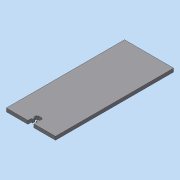
# Autodesk Inventor part: Y-Shafts-Holder_Side
Saved by Autodesk Inventor 2016 SP1 (Build 200210100, 210)
## iProperties
Created: 2016-01-21
Part Number: Y-Shafts-Holder_Side
Material: Generic
Document SubType Name: Modeling
Designer: Mohamed A.
Density: 1 g/cm^3
Appearance: Default
Author: Mohamed A.
Autodesk Inventor part; units mm, degrees
ref_plane "YZ Plane" through (0, 0, 0) normal (1, 0, 0) x (0, 1, 0)
ref_plane "XZ Plane" through (0, 0, 0) normal (0, 1, 0) x (-1, 0, 0)
ref_plane "XY Plane" through (0, 0, 0) normal (0, 0, 1) x (1, 0, 0)
sketch "Sketch1" plane through (0, 0, 0) normal (0, 0, 1) x (1, 0, 0)
  line L0 (-21.5, 51.7145) -> (21.5, 51.7145)
  line L1 (21.5, 51.7145) -> (21.5, -51.7145)
  line L2 (-21.5, -51.7145) -> (-21.5, 51.7145)
  line L3 (5.5, -51.7145) -> (5.5, -48.7145)
  line L4 (1.5, -46.7145) -> (2.65, -46.7145)
  line L5 (2.65, -46.7145) -> (2.65, -44.3145)
  line L6 (2.65, -44.3145) -> (1.5, -44.3145)
  line L7 (1.5, -44.3145) -> (1.5, -43.7145)
  line L8 (1.5, -43.7145) -> (-1.5, -43.7145)
  line L9 (-1.5, -43.7145) -> (-1.5, -44.3145)
  line L10 (-1.5, -44.3145) -> (-2.65, -44.3145)
  line L11 (-2.65, -44.3145) -> (-2.65, -46.7145)
  line L12 (-2.65, -46.7145) -> (-1.5, -46.7145)
  line L13 (-5.5, -48.7145) -> (-5.5, -51.7145)
  line L14 (1.5, -46.7145) -> (1.5, -48.7145)
  line L15 (1.5, -48.7145) -> (5.5, -48.7145)
  line L16 (-1.5, -46.7145) -> (-1.5, -48.7145)
  line L17 (-1.5, -48.7145) -> (-5.5, -48.7145)
  line L18 (21.5, -51.7145) -> (13.5, -51.7145)
  line L19 (-5.5, -51.7145) -> (-21.5, -51.7145)
  line L20 (-30.1, 0) -> (30.1, 0) construction
  line L21 (0, -72.4008) -> (0, 72.4004) construction
  line L22 (13.5, 44.7145) -> (13.5, 51.7145) projected
  line L23 (13.5, 51.7145) -> (10.5, 51.7145) projected
  line L24 (10.5, 44.7145) -> (10.5, 51.7145) projected
  line L25 (13.5, 44.7145) -> (10.5, 44.7145) projected
  line L26 (13.5, -4.1443) -> (13.5, 18.7145) projected
  line L27 (13.5, 18.7145) -> (10.5, 18.7145) projected
  line L28 (10.5, -4.1443) -> (10.5, 18.7145) projected
  line L29 (13.5, -4.1443) -> (10.5, -4.1443) projected
  line L30 (13.5, -51.7149) -> (13.5, -30.1443) projected
  line L31 (13.5, -30.1443) -> (10.5, -30.1443) projected
  line L32 (10.5, -51.7149) -> (10.5, -30.1443) projected
  line L33 (13.5, -51.7149) -> (10.5, -51.7149) projected
  line L34 (16.5, 41.7145) -> (16.5, 34.3645) projected
  line L35 (16.5, 41.7145) -> (13.5, 41.7145) projected
  line L36 (13.5, 34.3645) -> (13.5, 41.7145) projected
  line L37 (16.5, 34.3645) -> (13.5, 34.3645) projected
  line L38 (16.5, 29.0645) -> (16.5, 21.7145) projected
  line L39 (16.5, 29.0645) -> (13.5, 29.0645) projected
  line L40 (13.5, 21.7145) -> (13.5, 29.0645) projected
  line L41 (16.5, 21.7145) -> (13.5, 21.7145) projected
  line L42 (16.5, -7.1443) -> (16.5, -14.4943) projected
  line L43 (16.5, -7.1443) -> (13.5, -7.1443) projected
  line L44 (13.5, -14.4943) -> (13.5, -7.1443) projected
  line L45 (16.5, -14.4943) -> (13.5, -14.4943) projected
  line L46 (16.5, -19.7943) -> (16.5, -27.1443) projected
  line L47 (16.5, -19.7943) -> (13.5, -19.7943) projected
  line L48 (13.5, -27.1443) -> (13.5, -19.7943) projected
  line L49 (16.5, -27.1443) -> (13.5, -27.1443) projected
  line L50 (-13.5, -19.7943) -> (-13.5, -27.1443) projected
  line L51 (-13.5, -19.7943) -> (-16.5, -19.7943) projected
  line L52 (-16.5, -27.1443) -> (-16.5, -19.7943) projected
  line L53 (-13.5, -27.1443) -> (-16.5, -27.1443) projected
  line L54 (-13.5, -7.1443) -> (-13.5, -14.4943) projected
  line L55 (-13.5, -7.1443) -> (-16.5, -7.1443) projected
  line L56 (-16.5, -14.4943) -> (-16.5, -7.1443) projected
  line L57 (-13.5, -14.4943) -> (-16.5, -14.4943) projected
  line L58 (-13.5, 29.0645) -> (-13.5, 21.7145) projected
  line L59 (-13.5, 29.0645) -> (-16.5, 29.0645) projected
  line L60 (-16.5, 21.7145) -> (-16.5, 29.0645) projected
  line L61 (-13.5, 21.7145) -> (-16.5, 21.7145) projected
  line L62 (-13.5, 41.7145) -> (-13.5, 34.3645) projected
  line L63 (-13.5, 41.7145) -> (-16.5, 41.7145) projected
  line L64 (-16.5, 34.3645) -> (-16.5, 41.7145) projected
  line L65 (-13.5, 34.3645) -> (-16.5, 34.3645) projected
  line L66 (16.5, 34.3645) -> (13.5, 29.0645) construction
  line L67 (13.5, 34.3645) -> (16.5, 29.0645) construction
  line L68 (13.5, -14.4943) -> (16.5, -19.7943) construction
  line L69 (16.5, -14.4943) -> (13.5, -19.7943) construction
  line L70 (-13.5, -14.4943) -> (-16.5, -19.7943) construction
  line L71 (-16.5, -14.4943) -> (-13.5, -19.7943) construction
  line L72 (-13.5, 34.3645) -> (-16.5, 29.0645) construction
  line L73 (-16.5, 34.3645) -> (-13.5, 29.0645) construction
  circle A0 centre (-15, 31.7145) radius 1.4
  circle A1 centre (15, 31.7145) radius 1.4
  circle A2 centre (15, -17.1443) radius 1.4
  circle A3 centre (-15, -17.1443) radius 1.4
  line L74 (13.5, -51.7145) -> (10.5, -51.7145)
  line L75 (10.5, -51.7145) -> (5.5, -51.7145)
  dimension "d0" = 43
  dimension "d12" = 3
  dimension "d13" = 5.3
  dimension "d15" = 2.4
  dimension "d19" = 3
  dimension "d20" = 5
  dimension "d21" = 8
  dimension "d25" = 103.429
  dimension "d26" = 2.8
  dimension "d27" = 2.8
  dimension "d28" = 2.8
  dimension "d29" = 2.8
  dimension "d30" = 5
  constraints: 60 end point, 11 parallel, 11 perpendicular, 8 point on line, 4 centre point, 4 collinear, 4 midpoint, 3 vertical, 1 horizontal, 6 other
  measures "d0" distance of L1.end L2.start
  measures "d12" distance between parallel lines of L9 L7
  measures "d13" distance between parallel lines of L11 L5
  measures "d15" distance of L4.end L5.end
  measures "d19" distance between parallel lines of L18 L15
  measures "d20" distance between parallel lines of L18 L4
  measures "d21" distance between parallel lines of L18 L8
  measures "d25" distance between parallel lines of L18 L0
  measures "d26" diameter of A0
  measures "d27" diameter of A1
  measures "d28" diameter of A2
  measures "d29" diameter of A3
  measures "d30" distance between parallel lines of L3 L32
extrude "Extrusion1" add sketch "Sketch1" along normal blind 3 contours L0 L24 L25 L22 L1 L18 L30 L31 L32 L75 L3 L15 L14 L4 L5 L6 L7 L8 L9 L10 L11 L12 L16 L17 L13 L19 L2
body "Solid1"
